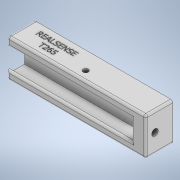
# Autodesk Inventor part: Part1
Saved by Autodesk Inventor 2021.4 (Build 254397000, 397)
## iProperties
Created: 2023-11-13
Part Number: Part1
Material: 一般
Document SubType Name: Modeling
Designer: ryusei
Density: 1 g/cm^3
Appearance: 既定
Author: ryusei
Autodesk Inventor part; units mm, degrees
ref_plane "YZ Plane" through (0, 0, 0) normal (1, 0, 0) x (0, 1, 0)
ref_plane "XZ Plane" through (0, 0, 0) normal (0, 1, 0) x (-1, 0, 0)
ref_plane "XY Plane" through (0, 0, 0) normal (0, 0, 1) x (1, 0, 0)
sketch "スケッチ1" plane through (0, 0, 0) normal (0, 0, 1) x (1, 0, 0)
  line L0 (-64, 17.5) -> (64, 17.5)
  line L1 (64, 17.5) -> (64, -17.5)
  line L2 (64, -17.5) -> (-64, -17.5)
  line L3 (-64, -17.5) -> (-64, 17.5)
  line L4 (-64, 17.5) -> (64, -17.5) construction
  line L5 (64, 17.5) -> (-64, -17.5) construction
  point P0 (0, 0)
  dimension "d0" = 128
  dimension "d1" = 35
  constraints: 12 end point, 2 midpoint, 2 parallel, 1 horizontal, 1 perpendicular
  measures "d0" distance of L1.end L2.end
  measures "d1" distance of L0.end L1.end
extrude "押し出し1" add sketch "スケッチ1" along normal blind 25
sketch "スケッチ3" plane through (-64, -17.5, 0) normal (-1, 0, 0) x (0, 0, 1)
  line L0 (9, 30.5) -> (23, 30.5)
  line L1 (23, 30.5) -> (23, 4.5)
  line L2 (23, 4.5) -> (9, 4.5)
  line L3 (9, 4.5) -> (9, 30.5)
  line L4 (0, 0) -> (25, 0) projected
  line L5 (25, 35) -> (25, 0) projected
  point P0 (0, 17.5)
  dimension "d8" = 14
  dimension "d9" = 26
  dimension "d10" = 4.5
  dimension "d11" = 2
  constraints: 8 end point, 2 parallel, 1 horizontal, 1 perpendicular
  measures "d8" distance of L1.end L2.end
  measures "d9" distance of L0.end L1.end
  measures "d10" distance between parallel lines of L4 L2
  measures "d11" distance between parallel lines of L5 L1
extrude "押し出し2" cut sketch "スケッチ3" against normal blind 118
sketch "スケッチ6" plane through (64, -17.5, 0) normal (1, 0, 0) x (0, 0, -1)
  line L0 (0, 0) -> (-25, 0) projected
  line L1 (0, 0) -> (0, 35) projected
  line L2 (-25, 0) -> (-25, 35) projected
  point P0 (0, 17.5)
  point P1 (-16.5, 17.5)
  dimension "d27" = 17.5
  dimension "d46" = 8.5
  measures "d27" distance from line of L0 point (-16.5, 17.5)
  measures "d46" distance from line of L2 point (-16.5, 17.5)
hole "穴2" at (64, 0, 16.5) direction (-1, 0, 0) diameter 6 end through all
sketch "スケッチ7" plane through (-64, 17.5, 0) normal (0, 1, 0) x (1, 0, 0)
  line L0 (128, 0) -> (0, 0) projected
  line L1 (128, 0) -> (128, -25) projected
  line L2 (128, -25) -> (0, -25) projected
  point P0 (64, 0)
  point P1 (64, -16.5)
  dimension "d37" = 64
  dimension "d45" = 8.5
  measures "d37" distance from line of L1 point (64, -16.5)
  measures "d45" distance from line of L2 point (64, -16.5)
hole "穴3" at (0, 17.5, 16.5) direction (0, -1, 0) diameter 4.9 depth 8
sketch "スケッチ8" plane through (-64, -13, 9) normal (0, 0, 1) x (1, 0, 0)
  point P0 (64, 13)
  point P1 (29, 13)
  point P2 (99, 13)
  dimension "d47" = 35
  dimension "d48" = 35
  measures "d47" distance of point (29, 13) point (64, 13)
  measures "d48" distance of point (99, 13) point (64, 13)
hole "穴4" at (-35, 0, 9) at (35, 0, 9) direction (0, 0, -1) diameter 6 depth 15 counterbore diameter 10 counterbore depth 6
sketch "スケッチ12" plane through (0, 0, 25) normal (0, 0, 1) x (1, 0, 0)
  line L0 (-64, 13) -> (-64, -13) projected
  line L1 (-64, 9.5) -> (51, 9.5)
  line L2 (51, 9.5) -> (51, -9.5)
  line L3 (51, -9.5) -> (-64, -9.5)
  line L4 (-64, -9.5) -> (-64, 9.5)
  point P0 (0, 0)
  dimension "d67" = 115
  dimension "d68" = 19
  dimension "d69" = 9.5
  constraints: 8 end point, 2 parallel, 1 horizontal, 1 perpendicular, 1 point on line
  measures "d67" distance of L2.end L3.end
  measures "d68" distance of L1.end L2.end
  measures "d69" distance from line of L1 point (0, 0)
extrude "押し出し7" cut sketch "スケッチ12" against normal blind 3
fillet "フィレット3" radius 2 12 edges at (-64, 17.5, 12.5) (0, 17.5, 25) (-6.5, 9.5, 25) (64, 17.5, 12.5) (64, 0, 25) (64, -17.5, 12.5) (0, -17.5, 25) (-6.5, -9.5, 25) (51, 0, 25) (-64, -17.5, 12.5) (-64, 13.5, 25) (-64, -13.5, 25)
sketch "スケッチ13" plane through (-62, 17.5, 0) normal (0, 1, 0) x (1, 0, 0)
  line L0 (9.2499, -5.5133) -> (44.882, -5.5133) construction
  line L1 (44.882, -5.5133) -> (44.882, -18.9402) construction
  line L2 (44.882, -18.9402) -> (9.2499, -18.9402) construction
  line L3 (9.2499, -18.9402) -> (9.2499, -5.5133) construction
  line L4 (13.6259, -10.6025) -> (12.7629, -10.6025)
  line L5 (12.7629, -10.6025) -> (11.1826, -8.613)
  line L6 (11.1826, -8.613) -> (10.4209, -8.613)
  line L7 (10.4209, -8.613) -> (10.4209, -10.6025)
  line L8 (10.4209, -10.6025) -> (9.7564, -10.6025)
  line L9 (9.7564, -10.6025) -> (9.7564, -5.6025)
  line L10 (9.7564, -5.6025) -> (11.0449, -5.6025)
  spline S0 degree 2 poles (11.0449, -5.6025) (11.4744, -5.6025) (12.0538, -5.6957) (12.3172, -5.8658) knots 0 0 0 1 2 2 2
  spline S1 degree 2 poles (12.3172, -5.8658) (12.5805, -6.036) (12.8844, -6.5668) (12.8844, -6.9599) knots 0 0 0 1 2 2 2
  spline S2 degree 2 poles (12.8844, -6.9599) (12.8844, -7.5069) (12.3253, -8.2483) (11.8472, -8.4266) knots 0 0 0 1 2 2 2
  line L11 (11.8472, -8.4266) -> (13.6259, -10.6025)
  spline S3 degree 2 poles (12.1916, -7.0125) (12.1916, -6.7937) (12.0376, -6.4574) (11.8755, -6.348) knots 0 0 0 1 2 2 2
  spline S4 degree 2 poles (11.8755, -6.348) (11.7337, -6.2548) (11.3569, -6.1778) (11.0813, -6.1778) knots 0 0 0 1 2 2 2
  line L12 (11.0813, -6.1778) -> (10.4209, -6.1778)
  line L13 (10.4209, -6.1778) -> (10.4209, -8.0579)
  line L14 (10.4209, -8.0579) -> (11.0044, -8.0579)
  spline S5 degree 2 poles (11.0044, -8.0579) (11.292, -8.0579) (11.7499, -7.9566) (11.9079, -7.7986) knots 0 0 0 1 2 2 2
  spline S6 degree 2 poles (11.9079, -7.7986) (12.0538, -7.6608) (12.1916, -7.2718) (12.1916, -7.0125) knots 0 0 0 1 2 2 2
  line L15 (14.023, -10.6025) -> (14.023, -5.6025)
  line L16 (14.023, -5.6025) -> (17.151, -5.6025)
  line L17 (17.151, -5.6025) -> (17.151, -6.194)
  line L18 (17.151, -6.194) -> (14.6875, -6.194)
  line L19 (14.6875, -6.194) -> (14.6875, -7.5636)
  line L20 (14.6875, -7.5636) -> (16.9849, -7.5636)
  line L21 (16.9849, -7.5636) -> (16.9849, -8.1551)
  line L22 (16.9849, -8.1551) -> (14.6875, -8.1551)
  line L23 (14.6875, -8.1551) -> (14.6875, -10.0109)
  line L24 (14.6875, -10.0109) -> (17.151, -10.0109)
  line L25 (17.151, -10.0109) -> (17.151, -10.6025)
  line L26 (17.151, -10.6025) -> (14.023, -10.6025)
  line L27 (17.3415, -10.6025) -> (19.0271, -5.6025)
  line L28 (19.0271, -5.6025) -> (19.8455, -5.6025)
  line L29 (19.8455, -5.6025) -> (21.5311, -10.6025)
  line L30 (21.5311, -10.6025) -> (20.8301, -10.6025)
  line L31 (20.8301, -10.6025) -> (20.3763, -9.2046)
  line L32 (20.3763, -9.2046) -> (18.4679, -9.2046)
  line L33 (18.4679, -9.2046) -> (18.0141, -10.6025)
  line L34 (18.0141, -10.6025) -> (17.3415, -10.6025)
  line L35 (20.194, -8.6373) -> (19.4201, -6.2832)
  line L36 (19.4201, -6.2832) -> (18.6502, -8.6373)
  line L37 (18.6502, -8.6373) -> (20.194, -8.6373)
  line L38 (24.9023, -10.6025) -> (22.0052, -10.6025)
  line L39 (22.0052, -10.6025) -> (22.0052, -5.6025)
  line L40 (22.0052, -5.6025) -> (22.6697, -5.6025)
  line L41 (22.6697, -5.6025) -> (22.6697, -10.0109)
  line L42 (22.6697, -10.0109) -> (24.9023, -10.0109)
  line L43 (24.9023, -10.0109) -> (24.9023, -10.6025)
  spline S7 degree 2 poles (26.8188, -10.6916) (26.2758, -10.6916) (25.5141, -10.4647) (25.1778, -10.3026) knots 0 0 0 1 2 2 2
  line L44 (25.1778, -10.3026) -> (25.1778, -9.468)
  line L45 (25.1778, -9.468) -> (25.2264, -9.468)
  spline S8 degree 2 poles (25.2264, -9.468) (25.5546, -9.7759) (26.3852, -10.1163) (26.7702, -10.1163) knots 0 0 0 1 2 2 2
  spline S9 degree 2 poles (26.7702, -10.1163) (27.3212, -10.1163) (27.8844, -9.6584) (27.8844, -9.2816) knots 0 0 0 1 2 2 2
  spline S10 degree 2 poles (27.8844, -9.2816) (27.8844, -8.9817) (27.5886, -8.609) (27.2685, -8.5158) knots 0 0 0 1 2 2 2
  spline S11 degree 2 poles (27.2685, -8.5158) (27.0376, -8.4509) (26.6527, -8.3618) (26.365, -8.2889) knots 0 0 0 1 2 2 2
  spline S12 degree 2 poles (26.365, -8.2889) (26.1057, -8.22) (25.6964, -8.0133) (25.5384, -7.8472) knots 0 0 0 1 2 2 2
  spline S13 degree 2 poles (25.5384, -7.8472) (25.3844, -7.6811) (25.2142, -7.2354) (25.2142, -6.9436) knots 0 0 0 1 2 2 2
  spline S14 degree 2 poles (25.2142, -6.9436) (25.2142, -6.3359) (26.1624, -5.5133) (26.8958, -5.5133) knots 0 0 0 1 2 2 2
  spline S15 degree 2 poles (26.8958, -5.5133) (27.3172, -5.5133) (28.0627, -5.6795) (28.3828, -5.8375) knots 0 0 0 1 2 2 2
  line L46 (28.3828, -5.8375) -> (28.3828, -6.6316)
  line L47 (28.3828, -6.6316) -> (28.3342, -6.6316)
  spline S16 degree 2 poles (28.3342, -6.6316) (28.0951, -6.4128) (27.3496, -6.0887) (26.9403, -6.0887) knots 0 0 0 1 2 2 2
  spline S17 degree 2 poles (26.9403, -6.0887) (26.4784, -6.0887) (25.9071, -6.5222) (25.9071, -6.8748) knots 0 0 0 1 2 2 2
  spline S18 degree 2 poles (25.9071, -6.8748) (25.9071, -7.1908) (26.2434, -7.5676) (26.5595, -7.6527) knots 0 0 0 1 2 2 2
  spline S19 degree 2 poles (26.5595, -7.6527) (26.7702, -7.7094) (27.382, -7.8553) (27.5846, -7.9161) knots 0 0 0 1 2 2 2
  spline S20 degree 2 poles (27.5846, -7.9161) (28.0992, -8.0741) (28.5773, -8.7103) (28.5773, -9.1762) knots 0 0 0 1 2 2 2
  spline S21 degree 2 poles (28.5773, -9.1762) (28.5773, -9.472) (28.3382, -10.0393) (28.1235, -10.2378) knots 0 0 0 1 2 2 2
  spline S22 degree 2 poles (28.1235, -10.2378) (27.8844, -10.4566) (27.2766, -10.6916) (26.8188, -10.6916) knots 0 0 0 1 2 2 2
  line L48 (29.254, -10.6025) -> (29.254, -5.6025)
  line L49 (29.254, -5.6025) -> (32.382, -5.6025)
  line L50 (32.382, -5.6025) -> (32.382, -6.194)
  line L51 (32.382, -6.194) -> (29.9185, -6.194)
  line L52 (29.9185, -6.194) -> (29.9185, -7.5636)
  line L53 (29.9185, -7.5636) -> (32.2159, -7.5636)
  line L54 (32.2159, -7.5636) -> (32.2159, -8.1551)
  line L55 (32.2159, -8.1551) -> (29.9185, -8.1551)
  line L56 (29.9185, -8.1551) -> (29.9185, -10.0109)
  line L57 (29.9185, -10.0109) -> (32.382, -10.0109)
  line L58 (32.382, -10.0109) -> (32.382, -10.6025)
  line L59 (32.382, -10.6025) -> (29.254, -10.6025)
  line L60 (36.6891, -10.6025) -> (35.9436, -10.6025)
  line L61 (35.9436, -10.6025) -> (33.7313, -6.2913)
  line L62 (33.7313, -6.2913) -> (33.7313, -10.6025)
  line L63 (33.7313, -10.6025) -> (33.1113, -10.6025)
  line L64 (33.1113, -10.6025) -> (33.1113, -5.6025)
  line L65 (33.1113, -5.6025) -> (34.0554, -5.6025)
  line L66 (34.0554, -5.6025) -> (36.0692, -9.5611)
  line L67 (36.0692, -9.5611) -> (36.0692, -5.6025)
  line L68 (36.0692, -5.6025) -> (36.6891, -5.6025)
  line L69 (36.6891, -5.6025) -> (36.6891, -10.6025)
  spline S23 degree 2 poles (39.0959, -10.6916) (38.553, -10.6916) (37.7912, -10.4647) (37.4549, -10.3026) knots 0 0 0 1 2 2 2
  line L70 (37.4549, -10.3026) -> (37.4549, -9.468)
  line L71 (37.4549, -9.468) -> (37.5036, -9.468)
  spline S24 degree 2 poles (37.5036, -9.468) (37.8318, -9.7759) (38.6624, -10.1163) (39.0473, -10.1163) knots 0 0 0 1 2 2 2
  spline S25 degree 2 poles (39.0473, -10.1163) (39.5984, -10.1163) (40.1616, -9.6584) (40.1616, -9.2816) knots 0 0 0 1 2 2 2
  spline S26 degree 2 poles (40.1616, -9.2816) (40.1616, -8.9817) (39.8658, -8.609) (39.5457, -8.5158) knots 0 0 0 1 2 2 2
  spline S27 degree 2 poles (39.5457, -8.5158) (39.3147, -8.4509) (38.9298, -8.3618) (38.6421, -8.2889) knots 0 0 0 1 2 2 2
  spline S28 degree 2 poles (38.6421, -8.2889) (38.3828, -8.22) (37.9736, -8.0133) (37.8155, -7.8472) knots 0 0 0 1 2 2 2
  spline S29 degree 2 poles (37.8155, -7.8472) (37.6616, -7.6811) (37.4914, -7.2354) (37.4914, -6.9436) knots 0 0 0 1 2 2 2
  spline S30 degree 2 poles (37.4914, -6.9436) (37.4914, -6.3359) (38.4395, -5.5133) (39.1729, -5.5133) knots 0 0 0 1 2 2 2
  spline S31 degree 2 poles (39.1729, -5.5133) (39.5943, -5.5133) (40.3399, -5.6795) (40.66, -5.8375) knots 0 0 0 1 2 2 2
  line L72 (40.66, -5.8375) -> (40.66, -6.6316)
  line L73 (40.66, -6.6316) -> (40.6113, -6.6316)
  spline S32 degree 2 poles (40.6113, -6.6316) (40.3723, -6.4128) (39.6267, -6.0887) (39.2175, -6.0887) knots 0 0 0 1 2 2 2
  spline S33 degree 2 poles (39.2175, -6.0887) (38.7556, -6.0887) (38.1843, -6.5222) (38.1843, -6.8748) knots 0 0 0 1 2 2 2
  spline S34 degree 2 poles (38.1843, -6.8748) (38.1843, -7.1908) (38.5206, -7.5676) (38.8366, -7.6527) knots 0 0 0 1 2 2 2
  spline S35 degree 2 poles (38.8366, -7.6527) (39.0473, -7.7094) (39.6591, -7.8553) (39.8617, -7.9161) knots 0 0 0 1 2 2 2
  spline S36 degree 2 poles (39.8617, -7.9161) (40.3763, -8.0741) (40.8544, -8.7103) (40.8544, -9.1762) knots 0 0 0 1 2 2 2
  spline S37 degree 2 poles (40.8544, -9.1762) (40.8544, -9.472) (40.6154, -10.0393) (40.4006, -10.2378) knots 0 0 0 1 2 2 2
  spline S38 degree 2 poles (40.4006, -10.2378) (40.1616, -10.4566) (39.5538, -10.6916) (39.0959, -10.6916) knots 0 0 0 1 2 2 2
  line L74 (41.5311, -10.6025) -> (41.5311, -5.6025)
  line L75 (41.5311, -5.6025) -> (44.6591, -5.6025)
  line L76 (44.6591, -5.6025) -> (44.6591, -6.194)
  line L77 (44.6591, -6.194) -> (42.1956, -6.194)
  line L78 (42.1956, -6.194) -> (42.1956, -7.5636)
  line L79 (42.1956, -7.5636) -> (44.493, -7.5636)
  line L80 (44.493, -7.5636) -> (44.493, -8.1551)
  line L81 (44.493, -8.1551) -> (42.1956, -8.1551)
  line L82 (42.1956, -8.1551) -> (42.1956, -10.0109)
  line L83 (42.1956, -10.0109) -> (44.6591, -10.0109)
  line L84 (44.6591, -10.0109) -> (44.6591, -10.6025)
  line L85 (44.6591, -10.6025) -> (41.5311, -10.6025)
  line L86 (21.1036, -18.8348) -> (21.1036, -14.4264)
  line L87 (21.1036, -14.4264) -> (19.4262, -14.4264)
  line L88 (19.4262, -14.4264) -> (19.4262, -13.8348)
  line L89 (19.4262, -13.8348) -> (23.4456, -13.8348)
  line L90 (23.4456, -13.8348) -> (23.4456, -14.4264)
  line L91 (23.4456, -14.4264) -> (21.7681, -14.4264)
  line L92 (21.7681, -14.4264) -> (21.7681, -18.8348)
  line L93 (21.7681, -18.8348) -> (21.1036, -18.8348)
  line L94 (26.8937, -18.8348) -> (23.8103, -18.8348)
  line L95 (23.8103, -18.8348) -> (23.8103, -18.1258)
  spline S39 degree 2 poles (23.8103, -18.1258) (24.1425, -17.8138) (24.7341, -17.2344) (25.0177, -16.9224) knots 0 0 0 1 2 2 2
  spline S40 degree 2 poles (25.0177, -16.9224) (25.589, -16.2943) (26.0064, -15.5407) (26.0064, -15.1395) knots 0 0 0 1 2 2 2
  spline S41 degree 2 poles (26.0064, -15.1395) (26.0064, -14.9288) (25.8767, -14.6128) (25.7592, -14.5115) knots 0 0 0 1 2 2 2
  spline S42 degree 2 poles (25.7592, -14.5115) (25.6417, -14.4102) (25.3338, -14.3089) (25.1474, -14.3089) knots 0 0 0 1 2 2 2
  spline S43 degree 2 poles (25.1474, -14.3089) (24.9691, -14.3089) (24.6044, -14.3981) (24.4383, -14.4669) knots 0 0 0 1 2 2 2
  spline S44 degree 2 poles (24.4383, -14.4669) (24.2965, -14.5237) (24.0331, -14.6857) (23.9521, -14.7425) knots 0 0 0 1 2 2 2
  line L96 (23.9521, -14.7425) -> (23.9156, -14.7425)
  line L97 (23.9156, -14.7425) -> (23.9156, -14.0293)
  spline S45 degree 2 poles (23.9156, -14.0293) (24.1223, -13.928) (24.8638, -13.7295) (25.196, -13.7295) knots 0 0 0 1 2 2 2
  spline S46 degree 2 poles (25.196, -13.7295) (25.897, -13.7295) (26.6871, -14.471) (26.6871, -15.1031) knots 0 0 0 1 2 2 2
  spline S47 degree 2 poles (26.6871, -15.1031) (26.6871, -15.3989) (26.5493, -15.8932) (26.4278, -16.1039) knots 0 0 0 1 2 2 2
  spline S48 degree 2 poles (26.4278, -16.1039) (26.3062, -16.3227) (25.9537, -16.7522) (25.7592, -16.9588) knots 0 0 0 1 2 2 2
  spline S49 degree 2 poles (25.7592, -16.9588) (25.4432, -17.3032) (24.6693, -18.0407) (24.4383, -18.2554) knots 0 0 0 1 2 2 2
  line L98 (24.4383, -18.2554) -> (26.8937, -18.2554)
  line L99 (26.8937, -18.2554) -> (26.8937, -18.8348)
  spline S50 degree 2 poles (30.7228, -17.2141) (30.7228, -17.599) (30.4675, -18.2514) (30.2527, -18.4702) knots 0 0 0 1 2 2 2
  spline S51 degree 2 poles (30.2527, -18.4702) (30.0299, -18.7011) (29.4707, -18.9402) (29.1344, -18.9402) knots 0 0 0 1 2 2 2
  spline S52 degree 2 poles (29.1344, -18.9402) (28.7981, -18.9402) (28.243, -18.7133) (28.0323, -18.4864) knots 0 0 0 1 2 2 2
  spline S53 degree 2 poles (28.0323, -18.4864) (27.773, -18.2149) (27.4813, -17.3032) (27.4813, -16.6387) knots 0 0 0 1 2 2 2
  spline S54 degree 2 poles (27.4813, -16.6387) (27.4813, -15.9864) (27.7487, -14.937) (28.0283, -14.548) knots 0 0 0 1 2 2 2
  spline S55 degree 2 poles (28.0283, -14.548) (28.2997, -14.1671) (29.1587, -13.7417) (29.7219, -13.7417) knots 0 0 0 1 2 2 2
  spline S56 degree 2 poles (29.7219, -13.7417) (29.8881, -13.7417) (30.1798, -13.7741) (30.2892, -13.8105) knots 0 0 0 1 2 2 2
  line L100 (30.2892, -13.8105) -> (30.2892, -14.4548)
  line L101 (30.2892, -14.4548) -> (30.2608, -14.4548)
  spline S57 degree 2 poles (30.2608, -14.4548) (30.1677, -14.4062) (29.8273, -14.3211) (29.6328, -14.3211) knots 0 0 0 1 2 2 2
  spline S58 degree 2 poles (29.6328, -14.3211) (29.0088, -14.3211) (28.243, -15.1639) (28.1701, -15.9904) knots 0 0 0 1 2 2 2
  spline S59 degree 2 poles (28.1701, -15.9904) (28.4091, -15.8243) (28.9116, -15.642) (29.2114, -15.642) knots 0 0 0 1 2 2 2
  spline S60 degree 2 poles (29.2114, -15.642) (29.5031, -15.642) (29.9407, -15.7595) (30.1798, -15.9378) knots 0 0 0 1 2 2 2
  spline S61 degree 2 poles (30.1798, -15.9378) (30.4553, -16.1444) (30.7228, -16.7846) (30.7228, -17.2141) knots 0 0 0 1 2 2 2
  spline S62 degree 2 poles (30.042, -17.2425) (30.042, -16.9345) (29.88, -16.5172) (29.7017, -16.3713) knots 0 0 0 1 2 2 2
  spline S63 degree 2 poles (29.7017, -16.3713) (29.568, -16.266) (29.2357, -16.1971) (29.0615, -16.1971) knots 0 0 0 1 2 2 2
  spline S64 degree 2 poles (29.0615, -16.1971) (28.8265, -16.1971) (28.3848, -16.3389) (28.1701, -16.4726) knots 0 0 0 1 2 2 2
  spline S65 degree 2 poles (28.1701, -16.4726) (28.166, -16.5455) (28.1579, -16.6833) (28.1579, -16.7887) knots 0 0 0 1 2 2 2
  spline S66 degree 2 poles (28.1579, -16.7887) (28.1579, -17.3073) (28.3605, -17.9434) (28.5145, -18.1096) knots 0 0 0 1 2 2 2
  spline S67 degree 2 poles (28.5145, -18.1096) (28.6563, -18.2676) (28.9642, -18.3932) (29.1385, -18.3932) knots 0 0 0 1 2 2 2
  spline S68 degree 2 poles (29.1385, -18.3932) (29.5437, -18.3932) (30.042, -17.8178) (30.042, -17.2425) knots 0 0 0 1 2 2 2
  spline S69 degree 2 poles (34.3451, -17.2465) (34.3451, -17.6071) (34.1142, -18.223) (33.9035, -18.4499) knots 0 0 0 1 2 2 2
  spline S70 degree 2 poles (33.9035, -18.4499) (33.6928, -18.6768) (33.0647, -18.9402) (32.6758, -18.9402) knots 0 0 0 1 2 2 2
  spline S71 degree 2 poles (32.6758, -18.9402) (32.3192, -18.9402) (31.6223, -18.7822) (31.367, -18.6566) knots 0 0 0 1 2 2 2
  line L102 (31.367, -18.6566) -> (31.367, -17.9475)
  line L103 (31.367, -17.9475) -> (31.4156, -17.9475)
  spline S72 degree 2 poles (31.4156, -17.9475) (31.4926, -18.0042) (31.7803, -18.1501) (31.9545, -18.2149) knots 0 0 0 1 2 2 2
  spline S73 degree 2 poles (31.9545, -18.2149) (32.1531, -18.2838) (32.4813, -18.3608) (32.6879, -18.3608) knots 0 0 0 1 2 2 2
  spline S74 degree 2 poles (32.6879, -18.3608) (32.8905, -18.3608) (33.2714, -18.2149) (33.4091, -18.0569) knots 0 0 0 1 2 2 2
  spline S75 degree 2 poles (33.4091, -18.0569) (33.5348, -17.907) (33.6644, -17.5099) (33.6644, -17.2425) knots 0 0 0 1 2 2 2
  spline S76 degree 2 poles (33.6644, -17.2425) (33.6644, -16.975) (33.5185, -16.6347) (33.3808, -16.5212) knots 0 0 0 1 2 2 2
  spline S77 degree 2 poles (33.3808, -16.5212) (33.239, -16.3956) (32.8176, -16.2903) (32.5623, -16.2903) knots 0 0 0 1 2 2 2
  spline S78 degree 2 poles (32.5623, -16.2903) (32.2868, -16.2903) (31.7398, -16.3754) (31.5737, -16.4118) knots 0 0 0 1 2 2 2
  line L104 (31.5737, -16.4118) -> (31.5737, -13.8348)
  line L105 (31.5737, -13.8348) -> (34.3168, -13.8348)
  line L106 (34.3168, -13.8348) -> (34.3168, -14.4224)
  line L107 (34.3168, -14.4224) -> (32.2179, -14.4224)
  line L108 (32.2179, -14.4224) -> (32.2179, -15.7554)
  spline S79 degree 2 poles (32.2179, -15.7554) (32.3395, -15.7392) (32.5745, -15.7271) (32.6717, -15.7271) knots 0 0 0 1 2 2 2
  spline S80 degree 2 poles (32.6717, -15.7271) (33.0566, -15.7271) (33.5874, -15.8527) (33.8305, -16.0391) knots 0 0 0 1 2 2 2
  spline S81 degree 2 poles (33.8305, -16.0391) (34.0777, -16.2254) (34.3451, -16.7927) (34.3451, -17.2465) knots 0 0 0 1 2 2 2
  point P0 (62, 0)
  constraints: 2 other
extrude "押し出し8" cut sketch "スケッチ13" against normal blind 1
